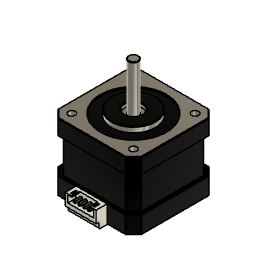
42步进电机 v8 (Autodesk Fusion 360 design; units mm, degrees)
Autodesk Fusion 360 part; units mm, degrees
sketch "草图1" plane through (0, 0, 0) normal (0, 0, 1) x (1, 0, 0)
  line L0 (17, 21) -> (-17, 21)
  line L1 (-21, 17) -> (-21, -17)
  line L2 (-17, -21) -> (17, -21)
  line L3 (21, -17) -> (21, 17)
  line L4 (21, 21) -> (-21, -21) construction
  line L5 (-21, 21) -> (21, -21) construction
  circle A0 centre (0, 0) radius 2.5
  circle A1 centre (0, 0) radius 11
  line L6 (-21, 17) -> (-17, 21)
  line L7 (17, 21) -> (21, 17)
  line L8 (-21, -17) -> (-17, -21)
  line L9 (17, -21) -> (21, -17)
  circle A2 centre (-15.5, 15.5) radius 1.75
  circle A3 centre (15.5, 15.5) radius 1.75
  circle A4 centre (-15.5, -15.5) radius 1.75
  circle A5 centre (15.5, -15.5) radius 1.75
  line L10 (-7.7552, -21.0001) -> (7.7448, -21.0001)
  line L11 (7.7448, -21.0001) -> (7.7448, -26.5001)
  line L12 (7.7448, -26.5001) -> (-7.7552, -26.5001)
  line L13 (-7.7552, -26.5001) -> (-7.7552, -21.0001)
  line L14 (-7.7552, -21.0001) -> (7.7448, -26.5001) construction
  line L15 (7.7448, -21.0001) -> (-7.7552, -26.5001) construction
  line L16 (-7.7552, -26.5001) -> (7.7448, -26.5001)
  line L17 (7.7448, -26.5001) -> (7.7448, -25.0966)
  line L18 (7.7448, -25.0966) -> (-7.7552, -25.0966)
  line L19 (-7.7552, -25.0966) -> (-7.7552, -26.5001)
  line L20 (-15.6226, 19.6226) -> (15.6139, 19.6226)
  line L21 (19.6139, 15.6226) -> (19.6139, -15.6139)
  line L22 (15.6139, -19.6139) -> (-15.6226, -19.6139)
  line L23 (-19.6226, -15.6139) -> (-19.6226, 15.6226)
  line L24 (-15.6226, 19.6226) -> (-19.6226, 15.6226)
  line L25 (-19.6226, -15.6139) -> (-15.6226, -19.6139)
  line L26 (15.6139, 19.6226) -> (19.6139, 15.6226)
  line L27 (19.6139, -15.6139) -> (15.6139, -19.6139)
  circle A6 centre (0, 0) radius 4.5517
  line L28 (-6.5008, -25.0966) -> (6.5009, -25.0966)
  line L29 (6.5009, -25.0966) -> (6.5009, -22.5381)
  line L30 (6.5009, -22.5381) -> (-6.5008, -22.5381)
  line L31 (-6.5008, -22.5381) -> (-6.5008, -25.0966)
  line L32 (-6.5008, -22.5381) -> (6.505, -22.5381)
  line L33 (6.505, -22.5381) -> (6.505, -26.5001)
  line L34 (6.505, -26.5001) -> (-6.5008, -26.5001)
  line L35 (-6.5008, -26.5001) -> (-6.5008, -22.5381)
  line L36 (-6.5008, -22.5381) -> (-4.5008, -22.5381)
  line L37 (-4.5008, -22.5381) -> (-4.5008, -25.0966)
  line L38 (-4.5008, -25.0966) -> (-6.5008, -25.0966)
  line L39 (-6.5008, -25.0966) -> (-6.5008, -22.5381)
  line L40 (6.5009, -22.5381) -> (4.5009, -22.5381)
  line L41 (4.5009, -22.5381) -> (4.5009, -25.0966)
  line L42 (4.5009, -25.0966) -> (6.5009, -25.0966)
  line L43 (6.5009, -25.0966) -> (6.5009, -22.5381)
  line L44 (-6.0016, -23.0172) -> (-4.9787, -23.0172)
  line L45 (-4.9787, -23.0172) -> (-4.9787, -25.5039)
  line L46 (-4.9787, -25.5039) -> (-6.0016, -25.5039)
  line L47 (-6.0016, -25.5039) -> (-6.0016, -23.0172)
  line L48 (5.001, -23.0096) -> (6.024, -23.0096)
  line L49 (6.024, -23.0096) -> (6.024, -25.5237)
  line L50 (6.024, -25.5237) -> (5.001, -25.5237)
  line L51 (5.001, -25.5237) -> (5.001, -23.0096)
  line L52 (-4.5008, -25.0966) -> (-6.5008, -25.0966)
  line L53 (-6.5008, -25.0966) -> (-6.5008, -26.5001)
  line L54 (-6.5008, -26.5001) -> (-4.5008, -26.5001)
  line L55 (-4.5008, -26.5001) -> (-4.5008, -25.0966)
  line L56 (4.5009, -25.0966) -> (6.505, -25.0966)
  line L57 (6.505, -25.0966) -> (6.505, -26.5001)
  line L58 (6.505, -26.5001) -> (4.5009, -26.5001)
  line L59 (4.5009, -26.5001) -> (4.5009, -25.0966)
  circle A7 centre (0, 0) radius 16.3262
  point P0 (-0.0052, -23.7501)
  point P1 (-19.6226, 19.6226)
  point P2 (19.6139, 19.6226)
  point P3 (19.6139, -19.6139)
  point P4 (-19.6226, -19.6139)
  dimension "d1" = 42
  dimension "d2" = 42
  dimension "d3" = 5
  dimension "d4" = 22
  dimension "d5" = 4
  dimension "d6" = 4
  dimension "d7" = 4
  dimension "d8" = 4
  dimension "d9" = 4
  dimension "d10" = 4
  dimension "d11" = 4
  dimension "d12" = 4
  dimension "d13" = 3.5
  dimension "d14" = 5.5
  dimension "d15" = 3.5
  dimension "d16" = 5.5
  dimension "d18" = 3.5
  dimension "d19" = 3.5
  dimension "d20" = 5.5
  dimension "d21" = 5.5
  dimension "d23" = 15.5
  dimension "d24" = 5.5
  dimension "d52" = 4
  dimension "d53" = 4
  dimension "d54" = 4
  dimension "d55" = 4
  dimension "d56" = 4
  dimension "d57" = 4
  dimension "d58" = 4
  dimension "d59" = 4
  dimension "d83" = 2
  dimension "d84" = 2
  dimension "d86" = 1.023
  constraint horizontal L0
  constraint perpendicular L0 L1
  constraint parallel L0 L2
  constraint parallel L1 L3
  constraint coincident L4 A0.centre
  constraint coincident L5 A0.centre
  constraint coincident A0.centre A1.centre
  constraint coincident L5.start L1
  constraint coincident L5.start L0
  constraint coincident L4.start L0
  constraint coincident L4.start L3
  constraint coincident L4.end L1
  constraint coincident L4.end L2
  constraint coincident L5.end L2
  constraint coincident L5.end L3
  constraint coincident L5 A2.centre
  constraint coincident L4 A3.centre
  constraint coincident L4 A4.centre
  constraint coincident L5 A5.centre
  constraint horizontal L10
  constraint perpendicular L10 L11
  constraint parallel L10 L12
  constraint parallel L11 L13
  constraint coincident L14 P0
  constraint coincident L15 P0
  constraint horizontal L16
  constraint vertical L17
  constraint horizontal L18
  constraint vertical L19
  constraint coincident L11 L17.end
  constraint horizontal L20
  constraint vertical L21
  constraint horizontal L22
  constraint vertical L23
  constraint coincident L5 P3
  constraint coincident L5 P1
  constraint coincident P1 L20
  constraint coincident P1 L23
  constraint coincident P4 L23
  constraint coincident P4 L22
  constraint coincident P2 L20
  constraint coincident P2 L21
  constraint coincident P3 L21
  constraint coincident P3 L22
  constraint horizontal L28
  constraint vertical L29
  constraint horizontal L30
  constraint vertical L31
  constraint coincident L18 L28.start
  constraint horizontal L32
  constraint vertical L33
  constraint horizontal L34
  constraint vertical L35
  constraint coincident L12 L33.end
  constraint horizontal L36
  constraint vertical L37
  constraint horizontal L38
  constraint vertical L39
  constraint horizontal L40
  constraint vertical L41
  constraint horizontal L42
  constraint vertical L43
  constraint horizontal L44
  constraint vertical L45
  constraint horizontal L46
  constraint vertical L47
  constraint horizontal L48
  constraint vertical L49
  constraint horizontal L50
  constraint vertical L51
  constraint horizontal L52
  constraint vertical L53
  constraint horizontal L54
  constraint vertical L55
  constraint horizontal L56
  constraint vertical L57
  constraint horizontal L58
  constraint vertical L59
  constraint concentric A0 A7
  constraint coincident L18 L56.end
  measures "d1" distance of L4.end L5.end
  measures "d2" distance of L5.start L4.end
  measures "d3" diameter of A0
  measures "d4" diameter of A1
  measures "d5" distance of L5.start L1.start
  measures "d6" distance of L5.start L0.end
  measures "d7" distance of L4.start L0.start
  measures "d8" distance of L4.start L3.end
  measures "d9" distance of L4.end L1.end
  measures "d10" distance of L4.end L2.start
  measures "d11" distance of L5.end L2.end
  measures "d12" distance of L5.end L3.start
  measures "d13" diameter of A2
  measures "d14" distance of L1 A2.centre
  measures "d15" diameter of A3
  measures "d16" distance of L3 A3.centre
  measures "d18" diameter of A4
  measures "d19" diameter of A5
  measures "d20" distance of L1 A4.centre
  measures "d21" distance of L3 A5.centre
  measures "d23" distance of L11.end L12.end
  measures "d24" distance of L10.end L11.end
  measures "d52" distance of P1 L20.start
  measures "d53" distance of P1 L23.end
  measures "d54" distance of P4 L23.start
  measures "d55" distance of P4 L22.end
  measures "d56" distance of P2 L20.end
  measures "d57" distance of P2 L21.start
  measures "d58" distance of P3 L21.end
  measures "d59" distance of P3 L22.start
  measures "d83" distance of L30.end L36.end
  measures "d84" distance of L29.end L40.end
  measures "d86" distance of L48.start L48.end
extrude "拉伸4" add sketch "草图1" against normal blind 34 contours L2 L10 L11 L13 L18 L30 L31 L32 L33 L35 L36 L39 L40 | L11 L12 L16 L17 L18 L33 L57 | L12 L13 L16 L18 L19 L35 L53 | L12 L16 L18 L28 L33 L34 L42 L49 L50 L51 L56 L57 L58 L59 | L18 L29 L32 L33 L43 L56 | L18 L28 L30 L31 L32 L35 L36 L37 L38 L39 L44 L45 L47 L52 | L12 L16 L18 L28 L34 L35 L38 L45 L46 L47 L52 L53 L54 L55 | L18 L28 L29 L30 L32 L40 L41 L42 L43 L48 L49 L51 L56 | L18 L28 L38 L44 L45 L47 L52 | L18 L28 L38 L45 L46 L47 L52 | L12 L16 L18 L28 L34 L55 L59 | L18 L28 L42 L49 L50 L51 L56 | L18 L28 L42 L48 L49 L51 L56 | L18 L28 L30 L32 L37 L41 makes body 1
extrude "拉伸5" cut sketch "草图1" against normal blind 25.8 contours L2 L10 L11 L13 L18 L30 L31 L32 L33 L35 L36 L39 L40 | L11 L12 L16 L17 L18 L33 L57 | L12 L13 L16 L18 L19 L35 L53 | L12 L16 L18 L28 L33 L34 L42 L49 L50 L51 L56 L57 L58 L59 | L18 L29 L32 L33 L43 L56 | L18 L28 L30 L31 L32 L35 L36 L37 L38 L39 L44 L45 L47 L52 | L12 L16 L18 L28 L34 L35 L38 L45 L46 L47 L52 L53 L54 L55 | L18 L28 L29 L30 L32 L40 L41 L42 L43 L48 L49 L51 L56 | L18 L28 L38 L44 L45 L47 L52 | L18 L28 L38 L45 L46 L47 L52 | L12 L16 L18 L28 L34 L55 L59 | L18 L28 L42 L49 L50 L51 L56 | L18 L28 L42 L48 L49 L51 L56 | L18 L28 L30 L32 L37 L41 bodies 1
extrude "拉伸8" cut sketch "草图1" against normal blind 34 contours L2 L10 L11 L13 L18 L30 L31 L32 L33 L35 L36 L39 L40 | L18 L29 L32 L33 L43 L56 | L18 L28 L30 L31 L32 L35 L36 L37 L38 L39 L44 L45 L47 L52 | L18 L28 L29 L30 L32 L40 L41 L42 L43 L48 L49 L51 L56 | L18 L28 L38 L44 L45 L47 L52 | L18 L28 L42 L48 L49 L51 L56 | L18 L28 L30 L32 L37 L41 bodies 1
extrude "拉伸9" cut sketch "草图1" against normal blind 35 contours L11 L12 L16 L17 L18 L33 L57 | L12 L13 L16 L18 L19 L35 L53 | L12 L16 L18 L28 L33 L34 L42 L49 L50 L51 L56 L57 L58 L59 | L12 L16 L18 L28 L34 L35 L38 L45 L46 L47 L52 L53 L54 L55 | L18 L28 L38 L45 L46 L47 L52 | L12 L16 L18 L28 L34 L55 L59 | L18 L28 L42 L49 L50 L51 L56 bodies 1
extrude "拉伸10" add sketch "草图1" against normal blind 34 contours L2 L10 L11 L13 L18 L30 L31 L32 L33 L35 L36 L39 L40 | L18 L29 L32 L33 L43 L56 | L18 L28 L30 L31 L32 L35 L36 L37 L38 L39 L44 L45 L47 L52 | L18 L28 L29 L30 L32 L40 L41 L42 L43 L48 L49 L51 L56 | L18 L28 L38 L44 L45 L47 L52 | L18 L28 L42 L48 L49 L51 L56 | L18 L28 L30 L32 L37 L41 bodies 1
extrude "拉伸11" add sketch "草图1" against normal blind 31 contours L11 L12 L16 L17 L18 L33 L57 | L12 L13 L16 L18 L19 L35 L53 | L12 L16 L18 L28 L33 L34 L42 L49 L50 L51 L56 L57 L58 L59 | L12 L16 L18 L28 L34 L35 L38 L45 L46 L47 L52 L53 L54 L55 | L18 L28 L38 L45 L46 L47 L52 | L12 L16 L18 L28 L34 L55 L59 | L18 L28 L42 L49 L50 L51 L56 bodies 1
extrude "拉伸12" cut sketch "草图1" against normal blind 25 contours L2 L10 L11 L13 L18 L30 L31 L32 L33 L35 L36 L39 L40 | L11 L12 L16 L17 L18 L33 L57 | L12 L13 L16 L18 L19 L35 L53 | L12 L16 L18 L28 L33 L34 L42 L49 L50 L51 L56 L57 L58 L59 | L18 L29 L32 L33 L43 L56 | L18 L28 L30 L31 L32 L35 L36 L37 L38 L39 L44 L45 L47 L52 | L12 L16 L18 L28 L34 L35 L38 L45 L46 L47 L52 L53 L54 L55 | L18 L28 L29 L30 L32 L40 L41 L42 L43 L48 L49 L51 L56 | L18 L28 L38 L44 L45 L47 L52 | L18 L28 L38 L45 L46 L47 L52 | L12 L16 L18 L28 L34 L55 L59 | L18 L28 L42 L49 L50 L51 L56 | L18 L28 L42 L48 L49 L51 L56 | L18 L28 L30 L32 L37 L41 bodies 1
extrude "拉伸13" add sketch "草图1" against normal blind 34 separate body contours L20 L21 L22 L23 L24 L25 L26 L27 | A7 makes body 2
extrude "拉伸14" add sketch "草图1" against normal blind 34 contours L0 L1 L2 L3 L6 L7 L8 L9 L10 bodies 2
extrude "拉伸15" cut sketch "草图1" against normal blind 25 contours L0 L1 L2 L3 L6 L7 L8 L9 L10 bodies 2
extrude "拉伸16" add sketch "草图1" against normal blind 8 contours L0 L1 L2 L3 L6 L7 L8 L9 L10 bodies 2
extrude "拉伸17" add sketch "草图1" against normal blind 34 contours A0 | A1 | A6 bodies 2
extrude "拉伸18" add sketch "草图1" along normal blind 2 contours A1 | A6 bodies 2
extrude "拉伸19" add sketch "草图1" along normal blind 24 contours A0 bodies 2
chamfer "倒角1" distance 0.3 angle 45 1 edges at (-2.3308, -0.904, 24) on bodies 2
extrude "拉伸20" cut sketch "草图1" along normal blind 2 contours A6 bodies 2
chamfer "倒角2" distance 0.3 angle 45 25 edges at (0, -21, 0) (21, 0, 0) (19, -19, 0) (19, 19, 0) (0, 21, 0) (-19, -19, 0) (-21, 0, 0) (-19, 19, 0) (-10.2556, -3.9778, 2) (-4.2437, 1.646, 2) (0, -21, -25) (-19, -19, -25) (-21, 0, -25) (19, 19, -25) (21, 0, -25) (19, -19, -25) (21, 0, -34) (19, -19, -34) (0, -21, -34) (0, 21, -25) (-19, 19, -25) (-19, 19, -34) (0, 21, -34) (19, 19, -34) (-21, 0, -34) on bodies 2
chamfer "倒角3" distance 0.3 angle 45 8 edges at (19, -19, -8) (21, 0, -8) (19, 19, -8) (0, -21, -8) (0, 21, -8) (-19, -19, -8) (-21, 0, -8) (-19, 19, -8) on bodies 2
fillet "圆角2" radius 0.3 24 edges at (19.6139, -15.6139, -16.5) (15.6139, -19.6139, -16.5) (21, -17, -29.5) (17, -21, -29.5) (19.6139, 15.6226, -16.5) (15.6139, 19.6226, -16.5) (21, 17, -29.5) (17, 21, -29.5) (-15.6226, 19.6226, -16.5) (-19.6226, 15.6226, -16.5) (-17, 21, -29.5) (-21, 17, -29.5) (-15.6226, -19.6139, -16.5) (-19.6226, -15.6139, -16.5) (-21, -17, -4) (-17, -21, -4) (-21, -17, -29.5) (-17, -21, -29.5) (17, -21, -4) (-21, 17, -4) (-17, 21, -4) (17, 21, -4) (21, 17, -4) (21, -17, -4) on bodies 2
extrude "拉伸21" cut sketch "草图1" against normal blind 29 contours L12 L16 L18 L28 L33 L34 L42 L49 L50 L51 L56 L57 L58 L59 | L18 L28 L30 L31 L32 L35 L36 L37 L38 L39 L44 L45 L47 L52 | L12 L16 L18 L28 L34 L35 L38 L45 L46 L47 L52 L53 L54 L55 | L18 L28 L29 L30 L32 L40 L41 L42 L43 L48 L49 L51 L56 | L18 L28 L38 L44 L45 L47 L52 | L18 L28 L38 L45 L46 L47 L52 | L12 L16 L18 L28 L34 L55 L59 | L18 L28 L42 L49 L50 L51 L56 | L18 L28 L42 L48 L49 L51 L56 | L18 L28 L30 L32 L37 L41 bodies 1
extrude "拉伸22" add sketch "草图1" against normal blind 25.5 contours L12 L16 L18 L28 L33 L34 L42 L49 L50 L51 L56 L57 L58 L59 | L18 L28 L30 L31 L32 L35 L36 L37 L38 L39 L44 L45 L47 L52 | L12 L16 L18 L28 L34 L35 L38 L45 L46 L47 L52 L53 L54 L55 | L18 L28 L29 L30 L32 L40 L41 L42 L43 L48 L49 L51 L56 bodies 1
extrude "拉伸23" cut sketch "草图1" against normal blind 25 contours L12 L16 L18 L28 L33 L34 L42 L49 L50 L51 L56 L57 L58 L59 | L18 L28 L30 L31 L32 L35 L36 L37 L38 L39 L44 L45 L47 L52 | L12 L16 L18 L28 L34 L35 L38 L45 L46 L47 L52 L53 L54 L55 | L18 L28 L29 L30 L32 L40 L41 L42 L43 L48 L49 L51 L56 bodies 1
sketch "草图3" plane through (0, 0, 0) normal (0, 1, 0) x (1, 0, 0)
  line L0 (-4.5008, 25) -> (-4.5008, 25.5)
  line L1 (-4.5008, 25.5) -> (-6.5008, 25.5)
  line L2 (-6.5008, 25.5) -> (-6.5008, 29)
  line L3 (-6.5008, 29) -> (6.5009, 29)
  line L4 (6.5009, 29) -> (6.5009, 25.5)
  line L5 (6.5009, 25.5) -> (4.5009, 25.5)
  line L6 (4.5009, 25.5) -> (4.5009, 25)
  line L7 (4.5009, 25) -> (-4.5008, 25)
  line L8 (-7.4903, 27.2703) -> (9.365, 27.2703) construction
  line L9 (-3.5502, 23.4652) -> (-3.5502, 30.4824) construction
  line L10 (-1.1725, 23.4237) -> (-1.1725, 30.4408) construction
  line L11 (1.2521, 23.5402) -> (1.2521, 30.5574) construction
  line L12 (3.5134, 23.4936) -> (3.5134, 30.4175) construction
  line L13 (-3.0502, 27.7703) -> (-4.0502, 27.7703)
  line L14 (-4.0502, 27.7703) -> (-4.0502, 26.7703)
  line L15 (-4.0502, 26.7703) -> (-3.0502, 26.7703)
  line L16 (-3.0502, 26.7703) -> (-3.0502, 27.7703)
  line L17 (-3.0502, 27.7703) -> (-4.0502, 26.7703) construction
  line L18 (-4.0502, 27.7703) -> (-3.0502, 26.7703) construction
  line L19 (-0.6725, 27.7703) -> (-1.6725, 27.7703)
  line L20 (-1.6725, 27.7703) -> (-1.6725, 26.7703)
  line L21 (-1.6725, 26.7703) -> (-0.6725, 26.7703)
  line L22 (-0.6725, 26.7703) -> (-0.6725, 27.7703)
  line L23 (-0.6725, 27.7703) -> (-1.6725, 26.7703) construction
  line L24 (-1.6725, 27.7703) -> (-0.6725, 26.7703) construction
  line L25 (1.7521, 27.7703) -> (0.7521, 27.7703)
  line L26 (0.7521, 27.7703) -> (0.7521, 26.7703)
  line L27 (0.7521, 26.7703) -> (1.7521, 26.7703)
  line L28 (1.7521, 26.7703) -> (1.7521, 27.7703)
  line L29 (1.7521, 27.7703) -> (0.7521, 26.7703) construction
  line L30 (0.7521, 27.7703) -> (1.7521, 26.7703) construction
  line L31 (4.0134, 27.7703) -> (3.0134, 27.7703)
  line L32 (3.0134, 27.7703) -> (3.0134, 26.7703)
  line L33 (3.0134, 26.7703) -> (4.0134, 26.7703)
  line L34 (4.0134, 26.7703) -> (4.0134, 27.7703)
  line L35 (4.0134, 27.7703) -> (3.0134, 26.7703) construction
  line L36 (3.0134, 27.7703) -> (4.0134, 26.7703) construction
  point P0 (-3.5502, 27.2703)
  point P1 (-1.1725, 27.2703)
  point P2 (1.2521, 27.2703)
  point P3 (3.5134, 27.2703)
  dimension "d92" = 1
  dimension "d93" = 1
  dimension "d94" = 1
  dimension "d95" = 1
  dimension "d96" = 1
  dimension "d97" = 1
  dimension "d98" = 1
  dimension "d99" = 1
  constraint perpendicular L4 L8
  constraint perpendicular L3 L10
  constraint perpendicular L3 L11
  constraint perpendicular L3 L12
  constraint equal L9 L10
  constraint equal L10 L11
  constraint parallel L9 L10
  constraint horizontal L13
  constraint perpendicular L13 L14
  constraint parallel L13 L15
  constraint parallel L14 L16
  constraint coincident L17 P0
  constraint coincident L18 P0
  constraint coincident L8 P0
  constraint coincident L9 P0
  constraint horizontal L19
  constraint perpendicular L19 L20
  constraint parallel L19 L21
  constraint parallel L20 L22
  constraint coincident L23 P1
  constraint coincident L24 P1
  constraint coincident L8 P1
  constraint coincident L10 P1
  constraint horizontal L25
  constraint perpendicular L25 L26
  constraint parallel L25 L27
  constraint parallel L26 L28
  constraint coincident L29 P2
  constraint coincident L30 P2
  constraint coincident L8 P2
  constraint coincident L11 P2
  constraint horizontal L31
  constraint perpendicular L31 L32
  constraint parallel L31 L33
  constraint parallel L32 L34
  constraint coincident L35 P3
  constraint coincident L36 P3
  constraint coincident L8 P3
  constraint coincident L12 P3
  measures "d92" distance of L14.end L15.end
  measures "d93" distance of L13.end L14.end
  measures "d94" distance of L20.end L21.end
  measures "d95" distance of L19.end L20.end
  measures "d96" distance of L26.end L27.end
  measures "d97" distance of L25.end L26.end
  measures "d98" distance of L32.end L33.end
  measures "d99" distance of L31.end L32.end
extrude "拉伸24" add sketch "草图3" against normal blind 26.4 contours L13 L14 L15 L16 | L19 L20 L21 L22 | L25 L26 L27 L28 | L31 L32 L33 L34 bodies 1
extrude "拉伸25" cut sketch "草图3" against normal blind 21 contours L13 L14 L15 L16 | L19 L20 L21 L22 | L25 L26 L27 L28 | L31 L32 L33 L34 bodies 1
chamfer "倒角4" distance 0.2 distance2 0.4 16 edges at (-3.5502, -26.4, -26.7703) (-3.0502, -26.4, -27.2703) (-3.5502, -26.4, -27.7703) (-4.0502, -26.4, -27.2703) (-1.1725, -26.4, -26.7703) (-0.6725, -26.4, -27.2703) (-1.1725, -26.4, -27.7703) (-1.6725, -26.4, -27.2703) (1.2521, -26.4, -27.7703) (0.7521, -26.4, -27.2703) (1.2521, -26.4, -26.7703) (1.7521, -26.4, -27.2703) (3.0134, -26.4, -27.2703) (3.5134, -26.4, -27.7703) (4.0134, -26.4, -27.2703) (3.5134, -26.4, -26.7703) measured on face at (-3.7169, -26.4, -27.437) measured on face at (-3.7169, -26.4, -27.437) measured on face at (-3.7169, -26.4, -27.437) measured on face at (-3.7169, -26.4, -27.437) measured on face at (-1.3392, -26.4, -27.437) measured on face at (-1.3392, -26.4, -27.437) measured on face at (-1.3392, -26.4, -27.437) measured on face at (-1.3392, -26.4, -27.437) measured on face at (1.4187, -26.4, -27.1036) measured on face at (1.4187, -26.4, -27.1036) measured on face at (1.4187, -26.4, -27.1036) measured on face at (1.4187, -26.4, -27.1036) measured on face at (3.3467, -26.4, -27.437) measured on face at (3.3467, -26.4, -27.437) measured on face at (3.3467, -26.4, -27.437) measured on face at (3.3467, -26.4, -27.437) on bodies 1
extrude "拉伸26" cut sketch "草图1" against normal blind 0.7 contours A7 bodies 2
fillet "圆角3" radius 0.5 1 edges at (-0.0052, -25.0966, -34) on bodies 1
fillet "圆角4" radius 0.25 1 edges at (-0.0052, -25.0966, -31) on bodies 1
chamfer "倒角5" distance 0.2 angle 45 1 edges at (-15.2214, 5.9038, 0) on bodies 2
equation "d6 = d5"
equation "d8 = d7"
equation "d10 = d9"
equation "d12 = d11"
equation "d53 = d52"
equation "d55 = d54"
equation "d57 = d56"
equation "d59 = d58"
